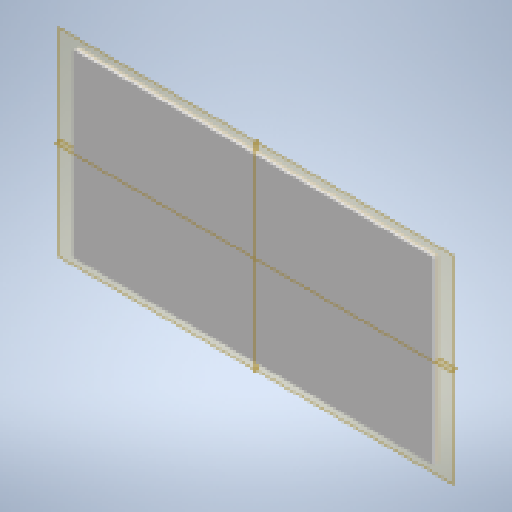
# Autodesk Inventor part: sessao_07_04_002_001
Saved by Autodesk Inventor 2026 (Build 300175000, 175)
## iProperties
Created: 2025-04-07
Part Number: sessao_07_04_002_001
Material: Generic
Document SubType Name: Modeling
Designer: Carlos Dias
Density: 1 g/cm^3
Appearance: Default
Author: Carlos Dias
Autodesk Inventor part; units mm, degrees
sketch "Sketch1" plane through (0, 0, 0) normal (0, 0, 1) x (1, 0, 0)
  line L0 (-250, 125) -> (250, 125)
  line L1 (250, 125) -> (250, -125)
  line L2 (250, -125) -> (-250, -125)
  line L3 (-250, -125) -> (-250, 125)
  line L4 (-250, 125) -> (250, -125) construction
  line L5 (250, 125) -> (-250, -125) construction
  point P0 (0, 0)
  point P1 (0, 0)
  dimension "d0" = 500
  dimension "d1" = 250
  constraints: 12 end point, 2 midpoint, 2 parallel, 1 coincident, 1 horizontal, 1 perpendicular
  measures "d0" distance of L0.start L0.end
  measures "d1" distance of L2.end L0.start
extrude "Extrusion1" add sketch "Sketch1" along normal mid plane 7
fillet "Fillet1" radius 2 4 edges at (250, 125, 0) (-250, 125, 0) (-250, -125, 0) (250, -125, 0)
sketch "Sketch2" plane through (0, 0, -3.5) normal (0, 0, -1) x (-1, 0, 0)
  line L0 (-102, -103) -> (-102, -57) projected
  line L1 (-102, -57) -> (-148, -57) projected
  line L2 (-148, -57) -> (-148, -103) projected
  line L3 (-148, -103) -> (-102, -103) projected
  line L4 (-105, -100) -> (-145, -100) projected
  line L5 (-145, -100) -> (-145, -60) projected
  line L6 (-145, -60) -> (-105, -60) projected
  line L7 (-105, -60) -> (-105, -100) projected
  line L8 (-101.5, -103.5) -> (-101.5, -56.5)
  line L9 (-101.5, -56.5) -> (-148.5, -56.5)
  line L10 (-148.5, -56.5) -> (-148.5, -103.5)
  line L11 (-148.5, -103.5) -> (-101.5, -103.5)
  line L12 (148, -103) -> (148, -57) projected
  line L13 (148, -57) -> (102, -57) projected
  line L14 (102, -57) -> (102, -103) projected
  line L15 (102, -103) -> (148, -103) projected
  line L16 (145, -100) -> (105, -100) projected
  line L17 (105, -100) -> (105, -60) projected
  line L18 (105, -60) -> (145, -60) projected
  line L19 (145, -60) -> (145, -100) projected
  line L20 (102, 103) -> (102, 57) projected
  line L21 (102, 57) -> (148, 57) projected
  line L22 (148, 57) -> (148, 103) projected
  line L23 (148, 103) -> (102, 103) projected
  line L24 (105, 100) -> (145, 100) projected
  line L25 (145, 100) -> (145, 60) projected
  line L26 (145, 60) -> (105, 60) projected
  line L27 (105, 60) -> (105, 100) projected
  line L28 (-148, 103) -> (-148, 57) projected
  line L29 (-148, 57) -> (-102, 57) projected
  line L30 (-102, 57) -> (-102, 103) projected
  line L31 (-102, 103) -> (-148, 103) projected
  line L32 (-145, 100) -> (-105, 100) projected
  line L33 (-105, 100) -> (-105, 60) projected
  line L34 (-105, 60) -> (-145, 60) projected
  line L35 (-145, 60) -> (-145, 100) projected
  line L36 (148.5, -103.5) -> (148.5, -56.5)
  line L37 (148.5, -56.5) -> (101.5, -56.5)
  line L38 (101.5, -56.5) -> (101.5, -103.5)
  line L39 (101.5, -103.5) -> (148.5, -103.5)
  line L40 (148.5, 56.5) -> (101.5, 56.5)
  line L41 (101.5, 56.5) -> (101.5, 103.5)
  line L42 (101.5, 103.5) -> (148.5, 103.5)
  line L43 (148.5, 103.5) -> (148.5, 56.5)
  line L44 (-101.5, 56.5) -> (-148.5, 56.5)
  line L45 (-148.5, 56.5) -> (-148.5, 103.5)
  line L46 (-148.5, 103.5) -> (-101.5, 103.5)
  line L47 (-101.5, 103.5) -> (-101.5, 56.5)
  point P0 (0, 0)
  dimension "d5" = 0.5
  constraints: 32 end point, 3 parallel, 12 other
  measures "d5" distance between parallel lines of L3 L11
extrude "Extrusion2" cut sketch "Sketch2" against normal blind 3.5 contours L3 L2 L1 L0 | L4 L5 L6 L7 | L11 L10 L9 L8 | L15 L14 L13 L12 | L16 L17 L18 L19 | L23 L22 L21 L20 | L24 L25 L26 L27 | L31 L30 L29 L28 | L32 L33 L34 L35 | L39 L38 L37 L36 | L40 L41 L42 L43 | L44 L45 L46 L47
body "Solid1"
